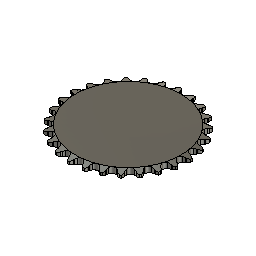
35Chain Sprocket Generator (Autodesk Fusion 360 design; units mm, degrees)
Autodesk Fusion 360 part; units mm, degrees
sketch "Teeth" plane through (0, 0, 0) normal (0, 0, 1) x (1, 0, 0)
  circle A0 centre (0, 0) radius 41.0232 construction
  line L0 (0, 41.0232) -> (-9.4606, 39.9174) construction
  arc A1 (-2.9536, 41.0687) -> (-2.0539, 39.4629) centre (3.2361, 43.4815) ccw
  line L1 (-2.9536, 41.0687) -> (-3.201, 41.7033)
  arc A2 (-3.201, 41.7033) -> (-4.4492, 43.4152) centre (-7.0639, 40.1975) ccw
  line L2 (0, 41.0232) -> (3.9262, 41.0232) construction
  line L3 (-2.9536, 41.0687) -> (3.2361, 43.4815) construction
  line L4 (3.2361, 43.4815) -> (0, 41.0232) construction
  line L5 (0, 41.0232) -> (0, 0) construction
  arc A3 (-2.0539, 39.4629) -> (0, 38.4438) centre (0, 41.0232) ccw
  arc A4 (4.4492, 43.4152) -> (3.201, 41.7033) centre (7.0639, 40.1975) ccw
  line L6 (2.9536, 41.0687) -> (3.201, 41.7033)
  arc A5 (2.0539, 39.4629) -> (2.9536, 41.0687) centre (-3.2361, 43.4815) ccw
  arc A6 (0, 38.4438) -> (2.0539, 39.4629) centre (0, 41.0232) ccw
  arc A7 (-4.4492, 43.4152) -> (-9.6393, 42.5647) centre (0, 0) ccw
  arc A8 (9.6393, 42.5647) -> (4.4492, 43.4152) centre (0, 0) ccw
  circle A9 centre (0, 0) radius 43.6426
  dimension "d11" = 82.0464
  dimension "d12" = 9.525
  dimension "d14" = 37.222
  dimension "d15" = 15.926
  dimension "d16" = 4.064
  dimension "d17" = 7.112
  dimension "d18" = 2.5794
  dimension "d20" = 43.6426
  dimension "d50" = 87.2851
  constraint coincident A0.centre L5.end
  constraint coincident A0 L0.start
  constraint coincident A0 L0.end
  constraint vertical A0.centre L0.start
  constraint tangent A1 L1
  constraint tangent L1 A2
  constraint tangent A0 L2
  constraint horizontal L2
  constraint perpendicular L1 L3
  constraint coincident L0 A2.centre
  constraint coincident A1.centre L3.end
  constraint coincident L5 A3.end
  constraint coincident L0 L2.start
  constraint coincident L0.start L2.start
  constraint tangent A1 A3
  constraint symmetric A1.end L5 A5.start
  constraint symmetric A1.start L5 L6.start
  constraint symmetric A1 L5 A5
  constraint symmetric L1.end L5 A4.end
  constraint symmetric A2 L5 A4
  constraint symmetric L5 A3.end A6.start
  constraint symmetric L5 A3 A6
  constraint vertical A0.centre A3.end
  constraint symmetric L5 A2.end A4.start
  constraint symmetric L5 A7.end A8.start
  constraint symmetric L5 A7 A8
  constraint coincident A4.start A8.end
  measures "d11" diameter of A0
  measures "d12" distance of L0.start L0.end
  measures "d14" angle of L2 L4
  measures "d15" angle of L3 L4
  measures "d16" distance of A1.centre L0.start
  measures "d17" distance of A2.centre L0.start
  measures "d18" radius of A3
  measures "d20" radius of A7
  measures "d50" diameter of A9
extrude "Extrude1" add sketch "Teeth" along normal mid plane 4.2926
extrude "Extrude3" cut sketch "Teeth" along normal through all and the other way through all contours A1 L1 A2 A3 A4 L6 A5 A6 A9
pattern_circular "C-Pattern1" count 27 over 360 about axis through (0, 0, 0) along (0, 0, 1) of "Extrude3"
sketch "Sketch4" plane through (0, 0, 0) normal (1, 0, 0) x (0, 1, 0)
  line L0 (-43.6426, 0.9525) -> (-38.4438, 2.1463)
  line L1 (-38.4438, 2.1463) -> (0, 2.1463)
  line L2 (-7.0051, 0) -> (0, 0) construction
  line L3 (-38.4438, -2.1463) -> (0, -2.1463)
  line L4 (-43.6426, -0.9525) -> (-38.4438, -2.1463)
  line L5 (0, -2.1463) -> (0, 2.1463)
  line L6 (-43.6426, 0.9525) -> (-43.6426, -0.9525)
  point P0 (-39.6283, 3.175)
  point P1 (-43.6426, 0)
  dimension "d49" = 38.4438
  dimension "d54" = 1.905
  dimension "d55" = 4.2926
  dimension "d56" = 43.6426
  constraint coincident L2.end origin
  constraint horizontal L1
  constraint horizontal L3
  constraint midpoint L5 L2.end
  constraint perpendicular L2 L6
  constraint midpoint L6 P1
  constraint vertical L5
  constraint equal L1 L3
  constraint horizontal L2.end P1
  measures "d49" distance of L3.end L3.start
  measures "d54" distance of L0.start L4.start
  measures "d55" distance of L1.end L3.end
  measures "d56" distance of L5 L6
revolve "Revolve1" cut sketch "Sketch4" angle 360 about axis through (0, 0, 1.75) along (0, 0, 1) keep common part
equation "p = 0.375 in" comment "0.25 for #25, 0.375 for #35"
equation "Dr = 0.2 in" comment "0.13 for #25, 0.2 for #35"
equation "Ds = 1.0005 * Dr + 0.003 in"
equation "n = 27" comment "Number of Teeth"
equation "PD = p / sin(( 180 / n ) * 1 deg)"
equation "A_angle = 35 deg + ( 60 / n ) * 1 deg"
equation "B_angle = 18 deg - ( 56 / n ) * 1 deg"
equation "ac = 0.8 * Dr"
equation "ab = 1.4 * Dr"
equation "OD = PD + 0.55 * p"
equation "d11 = PD"
equation "d12 = p"
equation "d14 = A_angle"
equation "d15 = B_angle"
equation "d16 = ac"
equation "d17 = ab"
equation "d18 = Ds / 2"
equation "d20 = OD / 2"
equation "d49 = ( PD - Ds ) / 2"
equation "d50 = OD"
equation "d52 = n"
equation "d56 = OD / 2"
